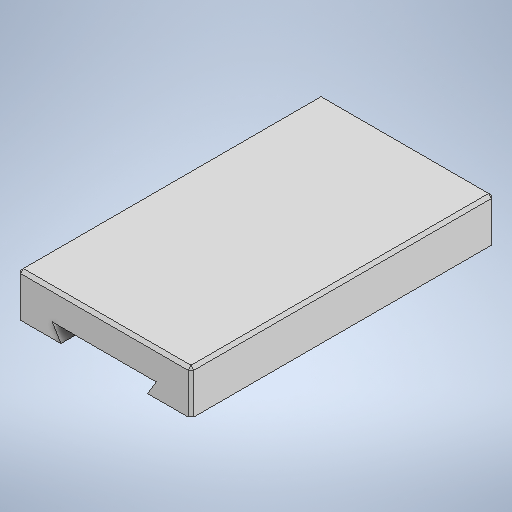
# Autodesk Inventor part: Cross Slide
Saved by Autodesk Inventor 2025 (Build 290162010, 162A)
## iProperties
Created: 2024-08-21
Part Number: Cross Slide
Material: Generic
Document SubType Name: Modeling
Designer: max_d
Density: 1 g/cm^3
Appearance: Default
Author: max_d
Autodesk Inventor part; units mm, degrees
ref_plane "YZ Plane" through (0, 0, 0) normal (1, 0, 0) x (0, 1, 0)
ref_plane "XZ Plane" through (0, 0, 0) normal (0, 1, 0) x (-1, 0, 0)
ref_plane "XY Plane" through (0, 0, 0) normal (0, 0, 1) x (1, 0, 0)
sketch "Sketch1" plane through (0, 0, 0) normal (0, 0, 1) x (1, 0, 0)
  line L0 (-60, 30) -> (60, 30)
  line L1 (60, 30) -> (60, 0)
  line L2 (60, 0) -> (30, 0)
  line L3 (30, 0) -> (36, 10)
  line L4 (36, 10) -> (-36, 10)
  line L5 (-36, 10) -> (-30, 0)
  line L6 (-30, 0) -> (-60, 0)
  line L7 (-60, 0) -> (-60, 30)
  line L8 (0, 0) -> (0, 10) construction
  line L9 (0, 10) -> (0, 30) construction
  dimension "d0" = 30
  dimension "d1" = 20
  dimension "d2" = 72
  dimension "d3" = 6
  dimension "d4" = 6
  dimension "d5" = 120
  dimension "d6" = 30
  constraints: 20 end point, 3 perpendicular, 2 midpoint, 2 point on line, 2 vertical, 1 horizontal, 1 parallel
  measures "d0" distance of L6.end L0.start
  measures "d1" distance between parallel lines of L0 L4
  measures "d2" distance of L3.end L4.end
  measures "d3" horizontal distance of L5.end L4.end
  measures "d4" horizontal distance of L3.end L2.end
  measures "d5" distance between parallel lines of L1 L7
  measures "d6" distance from line of L8.start L0
extrude "Extrusion1" add sketch "Sketch1" along normal blind 210
chamfer "Chamfer1" distance 2 angle 45 8 edges at (60, 15, 210) (60, 30, 105) (0, 30, 210) (-60, 15, 210) (-60, 30, 105) (-60, 15, 0) (0, 30, 0) (60, 15, 0)
body "Solid1"
